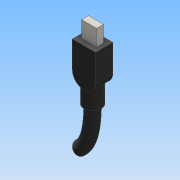
# Autodesk Inventor part: USB_cable
Saved by Autodesk Inventor 2016 (Build 200138000, 138)
## iProperties
Created: 2015-07-31
Part Number: USB_cable
Material: Generic
Document SubType Name: Modeling
Designer: Openlab
Density: 1 g/cm^3
Appearance: Rubber - Black
Author: Openlab
Autodesk Inventor part; units mm, degrees
ref_plane "YZ Plane" through (0, 0, 0) normal (1, 0, 0) x (0, 1, 0)
ref_plane "XZ Plane" through (0, 0, 0) normal (0, 1, 0) x (-1, 0, 0)
sketch "Sketch1" plane through (0, 0, 0) normal (0, 1, 0) x (-1, 0, 0)
  line L0 (8.25, -7) -> (-1.75, -7)
  line L1 (-1.75, -7) -> (-1.75, -18.5)
  line L2 (3.25, -23.5) -> (3.25, -23.5)
  line L3 (8.25, -18.5) -> (8.25, -7)
  line L4 (6.5, 0) -> (0, 0)
  line L5 (0, 0) -> (0, -7)
  line L6 (0, -7) -> (6.5, -7)
  line L7 (6.5, -7) -> (6.5, 0)
  line L8 (3.25, -4.5122) -> (3.25, -12.4364) construction
  arc A0 (3.25, -23.5) -> (8.25, -18.5) centre (3.25, -18.5) ccw
  arc A1 (-1.75, -18.5) -> (3.25, -23.5) centre (3.25, -18.5) ccw
  line L9 (3.25, -23.5) -> (3.25, -30.5)
  line L10 (3.25, -30.5) -> (3.25, -45.2683) construction
  line L11 (3.25, -45.2683) -> (8.7503, -49.7156) construction
  spline S0 degree 2 poles (3.25, -30.5) (3.25, -45.2683) (8.7503, -49.7156) knots 1 1 1 2 2 2
  point P0 (8.25, -23.5)
  dimension "d0" = 10
  dimension "d1" = 6.5
  dimension "d3" = 16.5
  dimension "d4" = 5
  dimension "d5" = 7
  dimension "d15" = 7
  constraints: 20 end point, 4 parallel, 4 point on circle, 4 tangent, 3 vertical, 2 centre point, 2 horizontal, 2 perpendicular, 2 point on line, 1 coincident, 1 collinear, 1 concentric, 5 other
  measures "d0" distance between parallel lines of L1 L3
  measures "d1" distance between parallel lines of L5 L7
  measures "d3" distance of point (8.25, -23.5) L0.start
  measures "d4" radius of A0
  measures "d5" distance of L6.end L4.start
  measures "d15" distance of L2.start L9.end
extrude "Extrusion1" add sketch "Sketch1" along normal mid plane 7.5 contours L3 A0 A1 L1 L0
extrude "Extrusion2" add sketch "Sketch1" along normal mid plane 3 contours L0 L5 L4 L7
ref_plane "Work Plane1" through (-3.25, 0, -23.5) normal (0, 0, -1) x (-1, 0, 0)
sketch "Sketch2" plane through (-3.25, 0, -23.5) normal (0, 0, -1) x (-1, 0, 0)
  circle A0 centre (0, 0) radius 3.75
  point P0 (-3.25, 0)
  dimension "d12" = 7.5
  constraints: 1 centre point
  measures "d12" diameter of A0
extrude "Extrusion3" add sketch "Sketch2" along normal blind 7 and the other way blind 2
sketch "Sketch3" plane through (-3.25, 0, -30.5) normal (0, 0, -1) x (-1, 0, 0)
  circle A0 centre (0, 0) radius 2.75
  point P0 (-3.25, 0)
  dimension "d18" = 5.5
  constraints: 1 centre point
  measures "d18" diameter of A0
sweep "Sweep1" add profiles "Sketch3" path "Sketch1" path curves L9 S0
body "Solid1"
